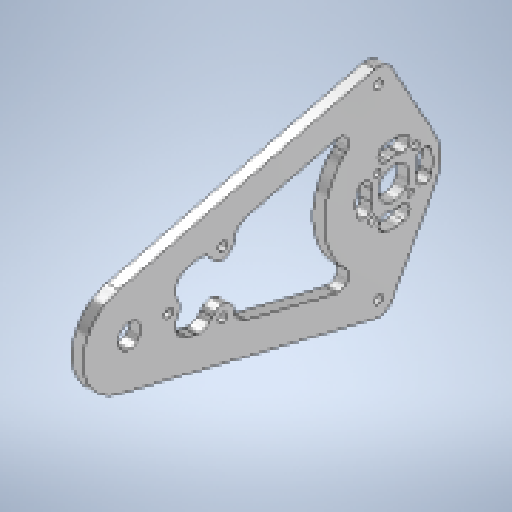
# Autodesk Inventor part: Upright - Motor
Saved by Autodesk Inventor 2023.4 (Build 274418000, 418)
## iProperties
Created: 2023-07-17
Part Number: Upright - Motor
Material: Aluminum 6061
Document SubType Name: Modeling
Designer: Nathan Cai
Mass: 72.2314 g
Surface Area: 155.597 cm^2
Volume: 26.7524 cm^3
Density: 2.7 g/cm^3
Appearance: Aluminum - Flat
C2C: 4.263 in
Bore: 0.375 in
S_Offset: 1.500 in
FrontOD: 1.500 in
Leg_Y_Back: 0.500 in
Leg_X_Back: 1.500 in
Leg_X_Front: 0.625 in
M2S: 0.250 in
Author: Nathan Cai
Autodesk Inventor part; units mm, degrees
ref_plane "YZ Plane" through (0, 0, 0) normal (1, 0, 0) x (0, 1, 0)
ref_plane "XZ Plane" through (0, 0, 0) normal (0, 1, 0) x (-1, 0, 0)
ref_plane "XY Plane" through (0, 0, 0) normal (0, 0, 1) x (1, 0, 0)
sketch "Sketch1" plane through (0, 0, 0) normal (1, 0, 0) x (0, 1, 0)
  circle A0 centre (0, 0) radius 19.05
  circle A1 centre (0, 0) radius 6.35
  circle A2 centre (0, 0) radius 25.4
  line L0 (0, 0) -> (0, 108.2802) construction
  circle A3 centre (0, 108.2802) radius 76.2 construction
  circle A4 centre (0, 108.2802) radius 4.7625
  line L1 (0, 6.35) -> (0, -38.1) construction
  line L2 (0, 6.35) -> (38.1, 6.35) construction
  circle A5 centre (38.1, 6.35) radius 1.7526
  circle A6 centre (38.1, 6.35) radius 6.35
  circle A7 centre (0, 108.2802) radius 15.875 construction
  circle A8 centre (0, 108.2802) radius 19.05
  line L3 (18.5007, 112.8219) -> (44.2669, 7.8639)
  line L4 (10.4489, 92.3515) -> (31.9331, 4.8361)
  line L5 (41.1454, 0.7779) -> (9.1361, -16.7163)
  arc A9 (21.9892, 12.7136) -> (29.2793, 15.6463) centre (25.425, 14.7001) ccw
  circle A10 centre (-38.1, 6.35) radius 1.7526
  circle A11 centre (-38.1, 6.35) radius 6.35
  line L6 (-18.5007, 112.8219) -> (-44.2669, 7.8639)
  line L7 (-10.4489, 92.3515) -> (-31.9331, 4.8361)
  line L8 (-41.1454, 0.7779) -> (-9.1361, -16.7163)
  arc A12 (-29.2793, 15.6463) -> (-21.9892, 12.7136) centre (-25.425, 14.7001) ccw
  circle A13 centre (12.7, 70.1802) radius 1.7526
  circle A14 centre (12.7, 70.1802) radius 4.7625
  circle A15 centre (-12.7, 70.1802) radius 1.7526
  circle A16 centre (-12.7, 70.1802) radius 4.7625
  circle A17 centre (0, 108.2802) radius 9.525 construction
  circle A18 centre (0, 92.4052) radius 1.7526
  circle A19 centre (0, 92.4052) radius 4.7625
  point P0 (-18.5007, 112.8219)
  point P1 (-9.1361, -16.7163)
  point P2 (-21.9892, 12.7136)
  point P3 (-16.5723, 67.4078)
  point P4 (-14.8483, 74.4306)
  point P5 (-10.4489, 92.3515)
  point P6 (14.8483, 74.4306)
  point P7 (16.5723, 67.4078)
  point P8 (3.8683, 89.6271)
  point P9 (-3.8683, 89.6271)
  dimension "d0" = 38.1
  dimension "d2" = 50.8
  dimension "d11" = 31.75
  dimension "d1" = 12.7
  dimension "d3" = 152.4
  dimension "C2C" = 108.2802
  dimension "Bore" = 9.525
  dimension "d6" = 44.45
  dimension "M2S" = 6.35
  dimension "S_Offset" = 38.1
  dimension "d9" = 3.5052
  dimension "d10" = 12.7
  dimension "FrontOD" = 38.1
  dimension "d13" = 7.9375
  dimension "d17" = 3.5052
  dimension "d18" = 9.525
  dimension "Leg_Y_Back" = 12.7
  dimension "Leg_X_Back" = 38.1
  dimension "d21" = 19.05
  dimension "d22" = 3.5052
  dimension "d51" = 9.525
  dimension "Leg_X_Front" = 15.875
  constraints: 18 end point, 17 centre point, 14 coincident, 13 symmetric about line, 12 point on circle, 5 point on line, 5 tangent, 1 parallel, 1 perpendicular, 1 vertical, 1 vertical alignment, 15 other
  measures "d1" diameter of A1
  measures "d3" diameter of A3
  measures "C2C" distance of L0.start L0.end
  measures "Bore" diameter of A4
  measures "d6" distance of L1.start L1.end
  measures "M2S" distance of point (0, 0) L1.start
  measures "S_Offset" distance of L1.start L2.end
  measures "d9" diameter of A5
  measures "d10" diameter of A6
  measures "FrontOD" diameter of A8
  measures "d13" diameter of A9
  measures "d17" diameter of A13
  measures "d18" diameter of A14
  measures "Leg_Y_Back" distance from line of L0 A14.centre
  measures "Leg_X_Back" vertical distance of A4.centre A14.centre
  measures "d21" diameter of A17
  measures "d22" diameter of A18
  measures "d51" diameter of A19
  measures "Leg_X_Front" distance of A4.centre A18.centre
extrude "Extrusion1" add sketch "Sketch1" along normal blind 4.7625 contours A0 | A0 L8 A2 L5 | L8 A11 L7 A12 A2 | A2 A9 L4 A6 L5 | A11 | A6 | L7 A11 L6 A8 A16 | L4 A14 A8 L3 A6 | A16 L7 | L7 A16 | A8 A19 | A14 L4 | L4 A14 | A19 A8 | A8 A19 picked at (14.284, 18.2012)
fillet "Fillet1" radius 6.35 8 edges at (2.3813, 10.4489, 92.3515) (2.3813, 14.8483, 74.4306) (2.3813, 16.5723, 67.4078) (2.3813, -10.4489, 92.3515) (2.3813, -14.8483, 74.4306) (2.3813, -16.5723, 67.4078) (2.3813, 3.8683, 89.6271) (2.3813, -3.8683, 89.6271)
sketch "Sketch5" plane through (4.7625, 0, 0) normal (-1, 0, 0) x (0, 0, 1)
  circle A0 centre (0, 0) radius 8 construction
  circle A1 centre (0, 0) radius 9.5 construction
  circle A2 centre (0, 0) radius 12.5 construction
  line L0 (0, 0) -> (0, 12.5) construction
  line L1 (0, 0) -> (8.8388, 8.8388) construction
  line L2 (0, 0) -> (-8.8388, 8.8388) construction
  circle A3 centre (6.7175, 6.7175) radius 1.5
  circle A4 centre (-8.8388, 8.8388) radius 1.5
  circle A5 centre (8.8388, -8.8388) radius 1.5
  circle A6 centre (-6.7175, -6.7175) radius 1.5
  circle A7 centre (0, 0) radius 12.7 construction
  arc A8 (3.287, 12.2673) -> (-3.287, 12.2673) centre (0, 0) ccw construction
  arc A9 (4.1088, 15.3341) -> (-4.1088, 15.3341) centre (0, 0) ccw
  arc A10 (2.4653, 9.2004) -> (-2.4653, 9.2004) centre (0, 0) ccw
  arc A11 (2.4653, 9.2004) -> (4.1088, 15.3341) centre (3.287, 12.2673) ccw
  arc A12 (-4.1088, 15.3341) -> (-2.4653, 9.2004) centre (-3.287, 12.2673) ccw
  line L3 (-3.287, 12.2673) -> (0, 0) construction
  line L4 (0, 0) -> (3.287, 12.2673) construction
  arc A13 (-9.2004, 2.4653) -> (-9.2004, -2.4653) centre (0, 0) ccw
  arc A14 (-9.2004, 2.4653) -> (-15.3341, 4.1088) centre (-12.2673, 3.287) ccw
  arc A15 (-15.3341, -4.1088) -> (-9.2004, -2.4653) centre (-12.2673, -3.287) ccw
  arc A16 (-15.3341, 4.1088) -> (-15.3341, -4.1088) centre (0, 0) ccw
  arc A17 (-12.2673, 3.287) -> (-12.2673, -3.287) centre (0, 0) ccw construction
  arc A18 (-2.4653, -9.2004) -> (2.4653, -9.2004) centre (0, 0) ccw
  arc A19 (-2.4653, -9.2004) -> (-4.1088, -15.3341) centre (-3.287, -12.2673) ccw
  arc A20 (4.1088, -15.3341) -> (2.4653, -9.2004) centre (3.287, -12.2673) ccw
  arc A21 (-4.1088, -15.3341) -> (4.1088, -15.3341) centre (0, 0) ccw
  arc A22 (-3.287, -12.2673) -> (3.287, -12.2673) centre (0, 0) ccw construction
  arc A23 (9.2004, -2.4653) -> (9.2004, 2.4653) centre (0, 0) ccw
  arc A24 (9.2004, -2.4653) -> (15.3341, -4.1088) centre (12.2673, -3.287) ccw
  arc A25 (15.3341, 4.1088) -> (9.2004, 2.4653) centre (12.2673, 3.287) ccw
  arc A26 (15.3341, -4.1088) -> (15.3341, 4.1088) centre (0, 0) ccw
  arc A27 (12.2673, -3.287) -> (12.2673, 3.287) centre (0, 0) ccw construction
  arc A28 (19.3929, 7.0584) -> (-1.7987, 20.559) centre (0, 0) ccw construction
  arc A29 (22.3764, 8.1444) -> (-2.0754, 23.7219) centre (0, 0) ccw
  arc A30 (16.4094, 5.9725) -> (-1.522, 17.396) centre (0, 0) ccw
  arc A31 (16.4094, 5.9725) -> (22.3764, 8.1444) centre (19.3929, 7.0584) ccw
  arc A32 (-2.0754, 23.7219) -> (-1.522, 17.396) centre (-1.7987, 20.559) ccw
  line L5 (0, 0) -> (-1.7987, 20.559) construction
  line L6 (0, 0) -> (19.3929, 7.0584) construction
  line L7 (0, 0) -> (6.35, 0) construction
  circle A33 centre (0, 0) radius 6.35 projected
  arc A34 (-2.0754, -23.7219) -> (22.3764, -8.1444) centre (0, 0) ccw
  arc A35 (-1.522, -17.396) -> (16.4094, -5.9725) centre (0, 0) ccw
  arc A36 (22.3764, -8.1444) -> (16.4094, -5.9725) centre (19.3929, -7.0584) ccw
  arc A37 (-1.522, -17.396) -> (-2.0754, -23.7219) centre (-1.7987, -20.559) ccw
  circle A38 centre (0, 0) radius 16 construction
  point P0 (-12.5, 0)
  point P1 (0, -12.5)
  point P2 (12.5, 0)
  dimension "d57" = 19
  dimension "d66" = 25.4
  dimension "d56" = 16
  dimension "d58" = 25
  dimension "d59" = 45
  dimension "d60" = 3
  dimension "d61" = 3
  dimension "d64" = 360
  dimension "d67" = 6.35
  dimension "d68" = 30
  dimension "d69" = 30
  dimension "d72" = 360
  dimension "d74" = 20.6375
  dimension "d75" = 6.35
  dimension "d76" = 5
  dimension "d77" = 70
  dimension "d87" = 32
  constraints: 61 point on circle, 36 centre point, 16 end point, 8 coincident, 8 tangent, 6 symmetric about line, 1 horizontal, 1 horizontal alignment, 1 perpendicular, 1 point on line, 1 vertical, 74 other
  measures "d56" diameter of A0
  measures "d58" diameter of A2
  measures "d59" angle of L0 L1
  measures "d60" diameter of A3
  measures "d61" diameter of A4
  measures "d67" diameter of A12
  measures "d68" angle of L2 L3
  measures "d69" angle of L1 L4
  measures "d74" radius of A28
  measures "d75" diameter of A31
  measures "d76" angle of L0 L5
  measures "d77" angle of L0 L6
  measures "d87" diameter of A38
extrude "Extrusion6" cut sketch "Sketch5" along normal through all contours A3 | A4 | A5 | A6 | A11 A10 A12 A9 | A13 A15 A16 A14 | A18 A20 A21 A19 | A23 A25 A26 A24
body "Solid1"
